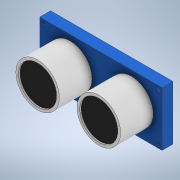
# Autodesk Inventor part: Ultraschallsensor
Saved by Autodesk Inventor 2021 (Build 250183000, 183)
## iProperties
Created: 2020-12-16
Part Number: Ultraschallsensor
Material: Generisch
Document SubType Name: Modeling
Designer: laure
Density: 1 g/cm^3
Appearance: Vorgabe
Author: laure
Autodesk Inventor part; units mm, degrees
ref_plane "YZ Plane" through (0, 0, 0) normal (1, 0, 0) x (0, 1, 0)
ref_plane "XZ Plane" through (0, 0, 0) normal (0, 1, 0) x (-1, 0, 0)
ref_plane "XY Plane" through (0, 0, 0) normal (0, 0, 1) x (1, 0, 0)
sketch "Skizze1" plane through (0, 0, 0) normal (0, 0, 1) x (1, 0, 0)
  line L0 (-22.5, 10) -> (22.5, 10)
  line L1 (22.5, 10) -> (22.5, -10)
  line L2 (22.5, -10) -> (-22.5, -10)
  line L3 (-22.5, -10) -> (-22.5, 10)
  line L4 (0, -14) -> (0, 14) projected
  line L5 (-31.5, 0) -> (31.5, 0) projected
  circle A0 centre (-11.25, 0) radius 8
  circle A1 centre (11.25, 0) radius 8
  circle A2 centre (-21.25, 8.75) radius 0.75
  circle A3 centre (21.25, 8.75) radius 0.75
  circle A4 centre (-21.25, -8.75) radius 0.75
  circle A5 centre (21.25, -8.75) radius 0.75
  circle A6 centre (-11.25, 0) radius 7
  circle A7 centre (11.25, 0) radius 7
  point P0 (0, 0)
  dimension "d0" = 20
  dimension "d1" = 45
  dimension "d2" = 16
  dimension "d3" = 11.25
  dimension "d4" = 1.5
  dimension "d5" = 1.25
  dimension "d6" = 1.25
  dimension "d11" = 1
  dimension "d12" = 1
  constraints: 8 centre point, 8 end point, 4 symmetric about line, 2 parallel, 1 horizontal, 1 perpendicular, 1 point on line, 6 other
  measures "d0" distance between parallel lines of L0 L2
  measures "d1" distance between parallel lines of L1 L3
  measures "d2" diameter of A0
  measures "d3" distance from line of A0.centre L4
  measures "d4" diameter of A2
  measures "d5" distance from line of L0 A2.centre
  measures "d6" distance from line of L3 A2.centre
  measures "d11" radial gap between concentric circles of A0 A6
  measures "d12" radial gap between concentric circles of A1 A7
extrude "Extrusion1" add sketch "Skizze1" against normal blind 4
extrude "Extrusion3" add sketch "Skizze1" along normal blind 12 contours A0 L5 A6 | L5 A6 A0 | A1 L5 A7 | L5 A7 A1
extrude "Extrusion4" add sketch "Skizze1" along normal blind 11.5 contours A6 L5 | L5 A6 | A7 L5 | L5 A7
